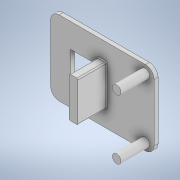
# Autodesk Inventor part: fleet
Saved by Autodesk Inventor 2020 (Build 240168000, 168)
## iProperties
Created: 2020-01-06
Part Number: fleet
Material: Generic
Document SubType Name: Modeling
Designer: my
Density: 1 g/cm^3
Appearance: Default
Author: my
Autodesk Inventor part; units mm, degrees
ref_plane "YZ Plane" through (0, 0, 0) normal (1, 0, 0) x (0, 1, 0)
ref_plane "XZ Plane" through (0, 0, 0) normal (0, 1, 0) x (-1, 0, 0)
ref_plane "XY Plane" through (0, 0, 0) normal (0, 0, 1) x (1, 0, 0)
sketch "Sketch1" plane through (0, 0, 0) normal (0, 0, 1) x (1, 0, 0)
  line L0 (-75, -65) -> (75, -65)
  line L1 (90, -50) -> (90, 50)
  line L2 (75, 65) -> (-75, 65)
  line L3 (-90, 50) -> (-90, -50)
  line L4 (-90, -65) -> (90, 65) construction
  line L5 (90, -65) -> (-90, 65) construction
  arc A0 (75, -65) -> (90, -50) centre (75, -50) ccw
  arc A1 (90, 50) -> (75, 65) centre (75, 50) ccw
  arc A2 (-75, 65) -> (-90, 50) centre (-75, 50) ccw
  arc A3 (-90, -50) -> (-75, -65) centre (-75, -50) ccw
  point P0 (0, 0)
  dimension "d0" = 180
  dimension "d1" = 130
  dimension "d9" = 15
  dimension "d10" = 15
  constraints: 12 end point, 8 point on circle, 8 point on line, 8 tangent, 4 centre point, 2 equal radius, 2 midpoint, 2 parallel, 1 horizontal, 1 perpendicular
  measures "d0" distance of L4.end L5.end
  measures "d1" distance of L5.start L4.end
  measures "d9" radius of A0
  measures "d10" radius of A1
extrude "Extrusion1" add sketch "Sketch1" along normal blind 7
sketch "Sketch3" plane through (0, 0, 7) normal (0, 0, 1) x (1, 0, 0)
  circle A0 centre (75, -52) radius 7.5
  circle A1 centre (75, 52) radius 7.5
  line L0 (7.5, 35) -> (-7.5, 35)
  line L1 (-7.5, 35) -> (-7.5, -35)
  line L2 (-7.5, -35) -> (7.5, -35)
  line L3 (7.5, -35) -> (7.5, 35)
  line L4 (7.5, 35) -> (-7.5, -35) construction
  line L5 (-7.5, 35) -> (7.5, -35) construction
  point P0 (0, 0)
  point P1 (0, 0)
  dimension "d11" = 15
  dimension "d12" = 104
  dimension "d13" = 52
  dimension "d14" = 75
  dimension "d15" = 15
  dimension "d16" = 70
  dimension "d17" = 7.5
  dimension "d18" = 35
  constraints: 12 end point, 2 centre point, 2 midpoint, 2 parallel, 1 equal radius, 1 horizontal, 1 perpendicular, 1 vertical alignment
  measures "d11" diameter of A0
  measures "d12" distance of A1.centre A0.centre
  measures "d13" vertical distance of point (0, 0) A0.centre
  measures "d14" horizontal distance of A0.centre point (0, 0)
  measures "d15" distance of L1.end L2.end
  measures "d16" distance of L0.end L1.end
  measures "d17" distance from line of point (0, 0) L3
  measures "d18" distance from line of L2 point (0, 0)
extrude "Extrusion2" add sketch "Sketch3" along normal blind 50
sketch "Sketch4" plane through (0, 0, 7) normal (0, 0, 1) x (1, 0, 0)
  line L0 (-15.5, 23) -> (-55.5, 23)
  line L1 (-55.5, 23) -> (-55.5, -23)
  line L2 (-55.5, -23) -> (-15.5, -23)
  line L3 (-15.5, -23) -> (-15.5, 23)
  line L4 (-15.5, 23) -> (-55.5, -23) construction
  line L5 (-55.5, 23) -> (-15.5, -23) construction
  line L6 (-7.5, -35) -> (-7.5, 35) projected
  point P0 (0, 0)
  point P1 (-35.5, 0)
  dimension "d21" = 46
  dimension "d22" = 40
  dimension "d25" = 28
  constraints: 12 end point, 2 midpoint, 2 parallel, 1 horizontal, 1 horizontal alignment, 1 perpendicular
  measures "d21" distance of L2.end L0.start
  measures "d22" distance of L1.end L2.end
  measures "d25" distance from line of L6 point (-35.5, 0)
extrude "Extrusion3" cut sketch "Sketch4" against normal mid plane 50
fillet "Fillet1" radius 2 8 edges at (0, 35, 7) (7.5, 0, 7) (7.5, 35, 32) (-7.5, 35, 32) (-7.5, 0, 7) (-7.5, -35, 32) (0, -35, 7) (7.5, -35, 32)
body "Solid1"
